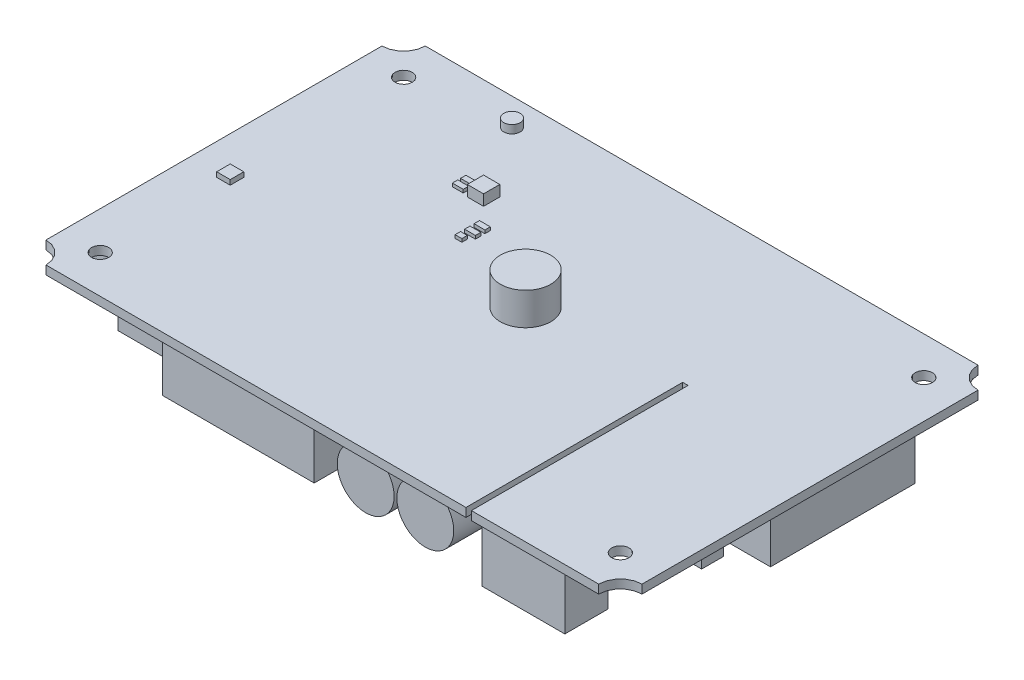
GridUp-PCB (Autodesk Fusion 360 design; units mm, degrees)
part number: 2026-09-14-08-15-55-205
Autodesk Fusion 360 part; units mm, degrees
sketch "Çizim181" plane through (0, 0, 0) normal (0, 0, 1) x (1, 0, 0)
  line L0 (0, 0) -> (110, 0)
  line L1 (110, 0) -> (110, 70)
  line L2 (110, 70) -> (0, 70)
  line L3 (0, 70) -> (0, 0)
extrude "Ekstrüzyon181" add sketch "Çizim181" along normal blind 1.6 makes body 1
fillet "Kavis6" radius 2 4 edges at (0, 70, 0.8) (110, 70, 0.8) (110, 0, 0.8) (0, 0, 0.8) on bodies 1
sketch "Çizim182" plane through (0, 0, 0) normal (0, 0, 1) x (1, 0, 0)
  circle A0 centre (7, 7) radius 1.6
  circle A1 centre (103, 7) radius 1.6
  circle A2 centre (7, 63) radius 1.6
  circle A3 centre (103, 63) radius 1.6
  line L0 (81.5, -1) -> (82.5, -1)
  line L1 (82.5, -1) -> (82.5, 40)
  line L2 (82.5, 40) -> (81.5, 40)
  line L3 (81.5, 40) -> (81.5, -1)
  circle A4 centre (0, 0) radius 4
  circle A5 centre (110, 0) radius 4
  circle A6 centre (0, 70) radius 4
  circle A7 centre (110, 70) radius 4
extrude "Ekstrüzyon182" cut sketch "Çizim182" along normal mid plane 10 bodies 1
ref_plane "WorkPlane168" through (0, 0, 1.6) normal (0, 0, 1) x (1, 0, 0)
sketch "Çizim183" plane through (0, 0, 1.6) normal (0, 0, 1) x (1, 0, 0)
  circle A0 centre (55, 37.5) radius 4.65
extrude "Ekstrüzyon183" add sketch "Çizim183" along normal blind 6 separate body makes body 2
ref_plane "WorkPlane169" through (0, 0, 1.6) normal (0, 0, 1) x (1, 0, 0)
sketch "Çizim184" plane through (0, 0, 1.6) normal (0, 0, 1) x (1, 0, 0)
  line L0 (5.75, 29.75) -> (8.25, 29.75)
  line L1 (8.25, 29.75) -> (8.25, 32.25)
  line L2 (8.25, 32.25) -> (5.75, 32.25)
  line L3 (5.75, 32.25) -> (5.75, 29.75)
extrude "Ekstrüzyon184" add sketch "Çizim184" along normal blind 0.9 separate body makes body 3
ref_plane "WorkPlane170" through (0, 0, 1.6) normal (0, 0, 1) x (1, 0, 0)
sketch "Çizim185" plane through (0, 0, 1.6) normal (0, 0, 1) x (1, 0, 0)
  circle A0 centre (25, 65) radius 1.5
extrude "Ekstrüzyon185" add sketch "Çizim185" along normal blind 1.5 separate body makes body 4
ref_plane "WorkPlane171" through (0, 0, 1.6) normal (0, 0, 1) x (1, 0, 0)
sketch "Çizim186" plane through (0, 0, 1.6) normal (0, 0, 1) x (1, 0, 0)
  line L0 (37.5, 45.5) -> (39.5, 45.5)
  line L1 (39.5, 45.5) -> (39.5, 46.5)
  line L2 (39.5, 46.5) -> (37.5, 46.5)
  line L3 (37.5, 46.5) -> (37.5, 45.5)
extrude "Ekstrüzyon186" add sketch "Çizim186" along normal blind 0.6 separate body makes body 5
ref_plane "WorkPlane172" through (0, 0, 1.6) normal (0, 0, 1) x (1, 0, 0)
sketch "Çizim187" plane through (0, 0, 1.6) normal (0, 0, 1) x (1, 0, 0)
  line L0 (37.5, 43.75) -> (39.5, 43.75)
  line L1 (39.5, 43.75) -> (39.5, 44.75)
  line L2 (39.5, 44.75) -> (37.5, 44.75)
  line L3 (37.5, 44.75) -> (37.5, 43.75)
extrude "Ekstrüzyon187" add sketch "Çizim187" along normal blind 0.6 separate body makes body 6
ref_plane "WorkPlane173" through (0, 0, 1.6) normal (0, 0, 1) x (1, 0, 0)
sketch "Çizim188" plane through (0, 0, 1.6) normal (0, 0, 1) x (1, 0, 0)
  line L0 (37.5, 42) -> (38.75, 42)
  line L1 (38.75, 42) -> (38.75, 43)
  line L2 (38.75, 43) -> (37.5, 43)
  line L3 (37.5, 43) -> (37.5, 42)
extrude "Ekstrüzyon188" add sketch "Çizim188" along normal blind 0.6 separate body makes body 7
ref_plane "WorkPlane174" through (0, 0, 1.6) normal (0, 0, 1) x (1, 0, 0)
sketch "Çizim189" plane through (0, 0, 1.6) normal (0, 0, 1) x (1, 0, 0)
  line L0 (29, 51.5) -> (31, 51.5)
  line L1 (31, 51.5) -> (31, 52.5)
  line L2 (31, 52.5) -> (29, 52.5)
  line L3 (29, 52.5) -> (29, 51.5)
extrude "Ekstrüzyon189" add sketch "Çizim189" along normal blind 0.6 separate body makes body 8
ref_plane "WorkPlane175" through (0, 0, 1.6) normal (0, 0, 1) x (1, 0, 0)
sketch "Çizim190" plane through (0, 0, 1.6) normal (0, 0, 1) x (1, 0, 0)
  line L0 (29, 50) -> (31, 50)
  line L1 (31, 50) -> (31, 51)
  line L2 (31, 51) -> (29, 51)
  line L3 (29, 51) -> (29, 50)
extrude "Ekstrüzyon190" add sketch "Çizim190" along normal blind 0.6 separate body makes body 9
ref_plane "WorkPlane176" through (0, 0, 1.6) normal (0, 0, 1) x (1, 0, 0)
sketch "Çizim191" plane through (0, 0, 1.6) normal (0, 0, 1) x (1, 0, 0)
  line L0 (32, 49.75) -> (35, 49.75)
  line L1 (35, 49.75) -> (35, 52.75)
  line L2 (35, 52.75) -> (32, 52.75)
  line L3 (32, 52.75) -> (32, 49.75)
extrude "Ekstrüzyon191" add sketch "Çizim191" along normal blind 2 separate body makes body 10
ref_plane "WorkPlane177" through (0, 0, 0) normal (0, 0, 1) x (1, 0, 0)
sketch "Çizim192" plane through (0, 0, 0) normal (0, 0, 1) x (1, 0, 0)
  line L0 (10, 40.8) -> (28, 40.8)
  line L1 (28, 40.8) -> (28, 60)
  line L2 (28, 60) -> (10, 60)
  line L3 (10, 60) -> (10, 40.8)
extrude "Ekstrüzyon192" add sketch "Çizim192" against normal blind 3.2 separate body makes body 11
ref_plane "WorkPlane178" through (0, 0, 0) normal (0, 0, 1) x (1, 0, 0)
sketch "Çizim193" plane through (0, 0, 0) normal (0, 0, 1) x (1, 0, 0)
  line L0 (64, 42) -> (95.7, 42)
  line L1 (95.7, 42) -> (95.7, 68.7)
  line L2 (95.7, 68.7) -> (64, 68.7)
  line L3 (64, 68.7) -> (64, 42)
extrude "Ekstrüzyon193" add sketch "Çizim193" against normal blind 21.8 separate body makes body 12
ref_plane "WorkPlane179" through (0, 0, 0) normal (0, 0, 1) x (1, 0, 0)
sketch "Çizim194" plane through (0, 0, 0) normal (0, 0, 1) x (1, 0, 0)
  line L0 (88, 22.25) -> (94.1, 22.25)
  line L1 (94.1, 22.25) -> (94.1, 25)
  line L2 (94.1, 25) -> (88, 25)
  line L3 (88, 25) -> (88, 22.25)
extrude "Ekstrüzyon194" add sketch "Çizim194" against normal blind 2.6 separate body makes body 13
ref_plane "WorkPlane180" through (0, 0, 0) normal (0, 0, 1) x (1, 0, 0)
sketch "Çizim195" plane through (0, 0, 0) normal (0, 0, 1) x (1, 0, 0)
  line L0 (96.5, 21.5) -> (103.5, 21.5)
  line L1 (103.5, 21.5) -> (103.5, 25.5)
  line L2 (103.5, 25.5) -> (96.5, 25.5)
  line L3 (96.5, 25.5) -> (96.5, 21.5)
extrude "Ekstrüzyon195" add sketch "Çizim195" against normal blind 8 separate body makes body 14
ref_plane "WorkPlane181" through (0, 0, 0) normal (0, 0, 1) x (1, 0, 0)
sketch "Çizim196" plane through (0, 0, 0) normal (0, 0, 1) x (1, 0, 0)
  line L0 (84, 0.5) -> (99.25, 0.5)
  line L1 (99.25, 0.5) -> (99.25, 8.5)
  line L2 (99.25, 8.5) -> (84, 8.5)
  line L3 (84, 8.5) -> (84, 0.5)
extrude "Ekstrüzyon196" add sketch "Çizim196" against normal blind 10 separate body makes body 15
ref_plane "WorkPlane182" through (0, 0, 0) normal (0, 0, 1) x (1, 0, 0)
sketch "Çizim197" plane through (0, 0, 0) normal (0, 0, 1) x (1, 0, 0)
  line L0 (70, 34) -> (76.5, 34)
  line L1 (76.5, 34) -> (76.5, 41)
  line L2 (76.5, 41) -> (70, 41)
  line L3 (70, 41) -> (70, 34)
extrude "Ekstrüzyon197" add sketch "Çizim197" against normal blind 1.7 separate body makes body 16
ref_plane "WorkPlane183" through (0, 0, 0) normal (0, 0, 1) x (1, 0, 0)
sketch "Çizim198" plane through (0, 0, 0) normal (0, 0, 1) x (1, 0, 0)
  line L0 (76.75, 39) -> (81, 39)
  line L1 (81, 39) -> (81, 41.65)
  line L2 (81, 41.65) -> (76.75, 41.65)
  line L3 (76.75, 41.65) -> (76.75, 39)
extrude "Ekstrüzyon198" add sketch "Çizim198" against normal blind 1.5 separate body makes body 17
ref_plane "WorkPlane184" through (0, 0, 0) normal (0, 0, 1) x (1, 0, 0)
sketch "Çizim199" plane through (0, 0, 0) normal (0, 0, 1) x (1, 0, 0)
  line L0 (76.75, 35) -> (81, 35)
  line L1 (81, 35) -> (81, 37.65)
  line L2 (81, 37.65) -> (76.75, 37.65)
  line L3 (76.75, 37.65) -> (76.75, 35)
extrude "Ekstrüzyon199" add sketch "Çizim199" against normal blind 1.5 separate body makes body 18
ref_plane "WorkPlane185" through (0, 0, 0) normal (0, 0, 1) x (1, 0, 0)
sketch "Çizim200" plane through (0, 0, 0) normal (0, 0, 1) x (1, 0, 0)
  line L0 (60.5, 44.5) -> (62.5, 44.5)
  line L1 (62.5, 44.5) -> (62.5, 45.5)
  line L2 (62.5, 45.5) -> (60.5, 45.5)
  line L3 (60.5, 45.5) -> (60.5, 44.5)
extrude "Ekstrüzyon200" add sketch "Çizim200" against normal blind 0.6 separate body makes body 19
ref_plane "WorkPlane186" through (0, 0, 0) normal (0, 0, 1) x (1, 0, 0)
sketch "Çizim201" plane through (0, 0, 0) normal (0, 0, 1) x (1, 0, 0)
  line L0 (77.5, 29.5) -> (79.5, 29.5)
  line L1 (79.5, 29.5) -> (79.5, 30.5)
  line L2 (79.5, 30.5) -> (77.5, 30.5)
  line L3 (77.5, 30.5) -> (77.5, 29.5)
extrude "Ekstrüzyon201" add sketch "Çizim201" against normal blind 0.6 separate body makes body 20
ref_plane "WorkPlane187" through (0, 0, 0) normal (0, 0, 1) x (1, 0, 0)
sketch "Çizim202" plane through (0, 0, 0) normal (0, 0, 1) x (1, 0, 0)
  line L0 (77.5, 28) -> (79.5, 28)
  line L1 (79.5, 28) -> (79.5, 29)
  line L2 (79.5, 29) -> (77.5, 29)
  line L3 (77.5, 29) -> (77.5, 28)
extrude "Ekstrüzyon202" add sketch "Çizim202" against normal blind 0.6 separate body makes body 21
ref_plane "WorkPlane188" through (0, 0, 0) normal (0, 0, 1) x (1, 0, 0)
sketch "Çizim203" plane through (0, 0, 0) normal (0, 0, 1) x (1, 0, 0)
  line L0 (46, 36) -> (48.5, 36)
  line L1 (48.5, 36) -> (48.5, 38)
  line L2 (48.5, 38) -> (46, 38)
  line L3 (46, 38) -> (46, 36)
extrude "Ekstrüzyon203" add sketch "Çizim203" against normal blind 1 separate body makes body 22
ref_plane "WorkPlane189" through (0, 0, 0) normal (0, 0, 1) x (1, 0, 0)
sketch "Çizim204" plane through (0, 0, 0) normal (0, 0, 1) x (1, 0, 0)
  line L0 (46, 31.5) -> (49, 31.5)
  line L1 (49, 31.5) -> (49, 34.5)
  line L2 (49, 34.5) -> (46, 34.5)
  line L3 (46, 34.5) -> (46, 31.5)
extrude "Ekstrüzyon204" add sketch "Çizim204" against normal blind 1.5 separate body makes body 23
ref_plane "WorkPlane190" through (0, 0, 0) normal (0, 0, 1) x (1, 0, 0)
sketch "Çizim205" plane through (0, 0, 0) normal (0, 0, 1) x (1, 0, 0)
  line L0 (52, 28) -> (54, 28)
  line L1 (54, 28) -> (54, 29)
  line L2 (54, 29) -> (52, 29)
  line L3 (52, 29) -> (52, 28)
extrude "Ekstrüzyon205" add sketch "Çizim205" against normal blind 0.6 separate body makes body 24
ref_plane "WorkPlane191" through (0, 0, 0) normal (0, 0, 1) x (1, 0, 0)
sketch "Çizim206" plane through (0, 0, 0) normal (0, 0, 1) x (1, 0, 0)
  line L0 (52, 30.5) -> (54, 30.5)
  line L1 (54, 30.5) -> (54, 31.5)
  line L2 (54, 31.5) -> (52, 31.5)
  line L3 (52, 31.5) -> (52, 30.5)
extrude "Ekstrüzyon206" add sketch "Çizim206" against normal blind 0.6 separate body makes body 25
ref_plane "WorkPlane192" through (0, 17.75, 0) normal (0, 1, 0) x (0, 0, 1)
sketch "Çizim207" plane through (0, 17.75, 0) normal (0, 1, 0) x (1, 0, 0)
  circle A0 centre (61, 5.25) radius 5.25
extrude "Ekstrüzyon207" add sketch "Çizim207" along normal mid plane 31.5 separate body makes body 26
sketch "Çizim208" plane through (0, 17.75, 0) normal (0, 1, 0) x (1, 0, 0)
  circle A0 centre (72, 5.25) radius 5.25
extrude "Ekstrüzyon208" add sketch "Çizim208" along normal mid plane 31.5 separate body makes body 27
ref_plane "WorkPlane193" through (0, 0, 0) normal (0, 0, 1) x (1, 0, 0)
sketch "Çizim209" plane through (0, 0, 0) normal (0, 0, 1) x (1, 0, 0)
  line L0 (41.25, 14) -> (46.25, 14)
  line L1 (46.25, 14) -> (46.25, 20)
  line L2 (46.25, 20) -> (41.25, 20)
  line L3 (41.25, 20) -> (41.25, 14)
extrude "Ekstrüzyon209" add sketch "Çizim209" against normal blind 1.5 separate body makes body 28
ref_plane "WorkPlane194" through (0, 0, 0) normal (0, 0, 1) x (1, 0, 0)
sketch "Çizim210" plane through (0, 0, 0) normal (0, 0, 1) x (1, 0, 0)
  line L0 (47.5, 15) -> (48.5, 15)
  line L1 (48.5, 15) -> (48.5, 17)
  line L2 (48.5, 17) -> (47.5, 17)
  line L3 (47.5, 17) -> (47.5, 15)
extrude "Ekstrüzyon210" add sketch "Çizim210" against normal blind 0.6 separate body makes body 29
ref_plane "WorkPlane195" through (0, 0, 0) normal (0, 0, 1) x (1, 0, 0)
sketch "Çizim211" plane through (0, 0, 0) normal (0, 0, 1) x (1, 0, 0)
  line L0 (1, 11) -> (9, 11)
  line L1 (9, 11) -> (9, 26.25)
  line L2 (9, 26.25) -> (1, 26.25)
  line L3 (1, 26.25) -> (1, 11)
extrude "Ekstrüzyon211" add sketch "Çizim211" against normal blind 10 separate body makes body 30
ref_plane "WorkPlane196" through (0, 0, 0) normal (0, 0, 1) x (1, 0, 0)
sketch "Çizim212" plane through (0, 0, 0) normal (0, 0, 1) x (1, 0, 0)
  line L0 (25, 14) -> (27, 14)
  line L1 (27, 14) -> (27, 15)
  line L2 (27, 15) -> (25, 15)
  line L3 (25, 15) -> (25, 14)
extrude "Ekstrüzyon212" add sketch "Çizim212" against normal blind 0.6 separate body makes body 31
ref_plane "WorkPlane197" through (0, 0, 0) normal (0, 0, 1) x (1, 0, 0)
sketch "Çizim213" plane through (0, 0, 0) normal (0, 0, 1) x (1, 0, 0)
  line L0 (28, 14) -> (30, 14)
  line L1 (30, 14) -> (30, 15)
  line L2 (30, 15) -> (28, 15)
  line L3 (28, 15) -> (28, 14)
extrude "Ekstrüzyon213" add sketch "Çizim213" against normal blind 0.6 separate body makes body 32
ref_plane "WorkPlane198" through (0, 0, 0) normal (0, 0, 1) x (1, 0, 0)
sketch "Çizim214" plane through (0, 0, 0) normal (0, 0, 1) x (1, 0, 0)
  line L0 (31, 14) -> (33, 14)
  line L1 (33, 14) -> (33, 15)
  line L2 (33, 15) -> (31, 15)
  line L3 (31, 15) -> (31, 14)
extrude "Ekstrüzyon214" add sketch "Çizim214" against normal blind 0.6 separate body makes body 33
ref_plane "WorkPlane199" through (0, 0, 0) normal (0, 0, 1) x (1, 0, 0)
sketch "Çizim215" plane through (0, 0, 0) normal (0, 0, 1) x (1, 0, 0)
  line L0 (34, 14) -> (36, 14)
  line L1 (36, 14) -> (36, 15)
  line L2 (36, 15) -> (34, 15)
  line L3 (34, 15) -> (34, 14)
extrude "Ekstrüzyon215" add sketch "Çizim215" against normal blind 0.6 separate body makes body 34
ref_plane "WorkPlane200" through (0, 0, 0) normal (0, 0, 1) x (1, 0, 0)
sketch "Çizim216" plane through (0, 0, 0) normal (0, 0, 1) x (1, 0, 0)
  line L0 (37, 13) -> (39, 13)
  line L1 (39, 13) -> (39, 15)
  line L2 (39, 15) -> (37, 15)
  line L3 (37, 15) -> (37, 13)
extrude "Ekstrüzyon216" add sketch "Çizim216" against normal blind 0.6 separate body makes body 35
ref_plane "WorkPlane201" through (0, 0, 0) normal (0, 0, 1) x (1, 0, 0)
sketch "Çizim217" plane through (0, 0, 0) normal (0, 0, 1) x (1, 0, 0)
  line L0 (25, 0.5) -> (53, 0.5)
  line L1 (53, 0.5) -> (53, 7.5)
  line L2 (53, 7.5) -> (25, 7.5)
  line L3 (25, 7.5) -> (25, 0.5)
extrude "Ekstrüzyon217" add sketch "Çizim217" against normal blind 9 separate body makes body 36
ref_plane "WorkPlane202" through (0, 0, 0) normal (0, 0, 1) x (1, 0, 0)
sketch "Çizim218" plane through (0, 0, 0) normal (0, 0, 1) x (1, 0, 0)
  line L0 (11, 6.25) -> (24, 6.25)
  line L1 (24, 6.25) -> (24, 11.25)
  line L2 (24, 11.25) -> (11, 11.25)
  line L3 (11, 11.25) -> (11, 6.25)
extrude "Ekstrüzyon218" add sketch "Çizim218" against normal blind 8.5 separate body makes body 37
equation "d749 = -( 3.2 mm )"
equation "d753 = -( 21.8 mm )"
equation "d757 = -( 2.6 mm )"
equation "d761 = -( 8 mm )"
equation "d765 = -( 10 mm )"
equation "d769 = -( 1.7 mm )"
equation "d773 = -( 1.5 mm )"
equation "d777 = -( 1.5 mm )"
equation "d781 = -( 0.6 mm )"
equation "d785 = -( 0.6 mm )"
equation "d789 = -( 0.6 mm )"
equation "d793 = -( 1 mm )"
equation "d797 = -( 1.5 mm )"
equation "d801 = -( 0.6 mm )"
equation "d805 = -( 0.6 mm )"
equation "d815 = -( 1.5 mm )"
equation "d819 = -( 0.6 mm )"
equation "d823 = -( 10 mm )"
equation "d827 = -( 0.6 mm )"
equation "d831 = -( 0.6 mm )"
equation "d835 = -( 0.6 mm )"
equation "d839 = -( 0.6 mm )"
equation "d843 = -( 0.6 mm )"
equation "d847 = -( 9 mm )"
equation "d851 = -( 8.5 mm )"
named bodies: "PCB", "MLX90640", "SHT31", "LED", "R_pullup1", "R_pullup2", "C_100n", "EN_RC1", "EN_RC2", "Reset", "ESP32-S3-WROOM-1U", "RAC05-05SK", "F1", "MOV", "Klemens 230V", "LDO SOT-223", "D1", "D2", "R_sarj", "Bolucu1", "Bolucu2", "Boost U7", "L_boost", "R_bal1", "R_bal2", "Superkap1", "Superkap2", "MAX3485", "R120", "Klemens RS-485", "R_burden1", "R_burden2", "R_burden3", "R_burden4", "R_bias", "Klemens CT", "Genisleme 2x5"
